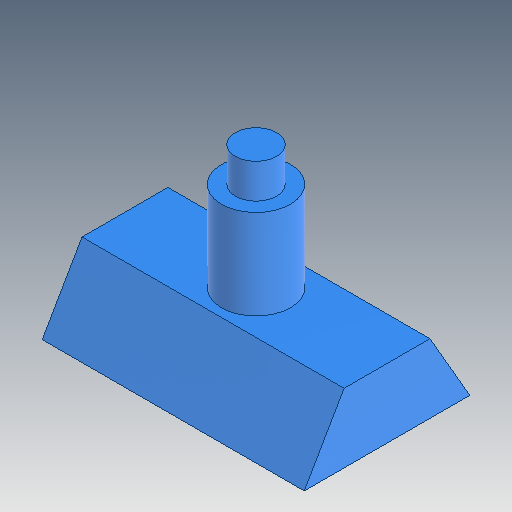
# Autodesk Inventor part: Sketch
Saved by Autodesk Inventor 2017 (Build 210142000, 142)
## iProperties
Created: 2020-02-29
Part Number: Sketch
Document SubType Name: Modeling
Designer: Administrator
Density: 1 g/cm^3
Material: Generic
Appearance: Cyan
Mass: 8.08846 g
Surface Area: 31.2997 cm^2
Volume: 8.08846 cm^3
Author: Administrator
Autodesk Inventor part; units mm, degrees
ref_plane "YZ Plane" through (0, 0, 0) normal (1, 0, 0) x (0, 1, 0)
ref_plane "XZ Plane" through (0, 0, 0) normal (0, 1, 0) x (-1, 0, 0)
ref_plane "XY Plane" through (0, 0, 0) normal (0, 0, 1) x (1, 0, 0)
sketch "Sketch4" plane through (0, 0, 0) normal (1, 0, 0) x (0, 1, 0)
  line L0 (0, 0) -> (0, -12)
  line L1 (0, -12) -> (10, -6.2265)
  line L2 (10, -6.2265) -> (10, 6.2265)
  line L3 (10, 6.2265) -> (0, 12)
  line L4 (0, 12) -> (0, 0)
  line L5 (0, 0) -> (10, 0)
  dimension "d31" = 60
  dimension "d32" = 60
  dimension "d33" = 10
  dimension "d34" = 12
  constraints: 12 end point, 2 collinear, 1 midpoint, 1 parallel, 1 perpendicular, 1 point on line, 1 vertical
  measures "d31" angle of L0 L1
  measures "d32" angle of L4 L3
  measures "d33" distance between parallel lines of L2 L0
  measures "d34" distance of L0.start L0.end
extrude "Extrusion3" add sketch "Sketch4" along normal mid plane 38
sketch "Sketch5" plane through (-19, 10, 6.2265) normal (0, 1, 0) x (1, 0, 0)
  circle A0 centre (19, 6.2265) radius 5
  dimension "d37" = 10
  constraints: 1 centre point, 1 coincident
  measures "d37" diameter of A0
extrude "Extrusion4" add sketch "Sketch5" along normal blind 13
sketch "Sketch6" plane through (0, 23, 0) normal (0, 1, 0) x (1, 0, 0)
  circle A0 centre (0, 0) radius 3
  point P0 (0, 0)
  dimension "d40" = 6
  constraints: 1 centre point, 1 coincident
  measures "d40" diameter of A0
extrude "Extrusion5" add sketch "Sketch6" along normal blind 5
body "Solid4"
